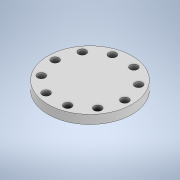
# Autodesk Inventor part: Крышка стакана
Saved by Autodesk Inventor 2021 (Build 250183000, 183)
## iProperties
Created: 2020-11-15
Part Number: Крышка стакана
Material: Типовые
Document SubType Name: Modeling
Designer: Тимоха
Density: 1 g/cm^3
Appearance: По умолчанию
Author: Тимоха
Autodesk Inventor part; units mm, degrees
ref_plane "YZ Plane" through (0, 0, 0) normal (1, 0, 0) x (0, 1, 0)
ref_plane "XZ Plane" through (0, 0, 0) normal (0, 1, 0) x (-1, 0, 0)
ref_plane "XY Plane" through (0, 0, 0) normal (0, 0, 1) x (1, 0, 0)
sketch "Эскиз1" plane through (0, 0, 0) normal (0, 0, 1) x (1, 0, 0)
  line L0 (0, 0) -> (78, 0)
  line L1 (78, 0) -> (78, 24)
  line L2 (78, 24) -> (120, 24)
  line L3 (120, 24) -> (120, 49)
  line L4 (120, 49) -> (0, 49)
  line L5 (65.5, 20.9431) -> (0, 20.9431)
  line L6 (0, 49) -> (0, 20.9431)
  line L7 (65.5, 20.9431) -> (65.5, 0)
  line L8 (65.5, 0) -> (73.5, 0)
  line L9 (73.5, 0) -> (78, 13.3185)
  line L10 (78, 14.7395) -> (75, 14.7395)
  line L11 (75, 14.7395) -> (75, 17.7395)
  line L12 (75, 17.7395) -> (78, 17.7395)
  dimension "d0" = 78
  dimension "d1" = 24
  dimension "d2" = 42
  dimension "d3" = 25
  dimension "d18" = 65.5
  dimension "d19" = 8
  dimension "d21" = 3
  dimension "d22" = 3
  constraints: 26 end point, 6 perpendicular, 5 point on line, 2 horizontal, 2 vertical
  measures "d0" distance of L0.start L0.end
  measures "d1" distance of L0.end L1.end
  measures "d2" distance of L1.end L2.end
  measures "d3" distance of L2.end L3.end
  measures "d18" distance of L5.start L5.end
  measures "d19" distance of L7.end L8.end
  measures "d21" distance of L10.start L10.end
  measures "d22" distance of L10.end L11.end
revolve "Вращение1" add sketch "Эскиз1" angle 360 about axis through (0, 49, 0) along (0, -1, 0) contours L7 L5 L6 L4 L3 L2 L1 L12 L11 L10 L9 L0
sketch "Эскиз2" plane through (0, 49, 0) normal (0, 1, 0) x (1, 0, 0)
  circle A0 centre (0, 0) radius 120 projected
  line L0 (120, 0) -> (99.5, 0)
  point P0 (0, 0)
  dimension "d7" = 20.5
  constraints: 2 end point, 1 horizontal, 1 horizontal alignment, 1 other
  measures "d7" distance of L0.start L0.end
hole "Отверстие1" at (99.5, 49, 0) direction (0, -1, 0) diameter 22 end through all
pattern_circular "Круговой массив1" count 10 over 360 about axis through (0, 10.4715, 0) along (0, -1, 0) of "Отверстие1"
fillet "Сопряжение1" radius 10 1 edges at (-65.5, 20.9431, 0)
